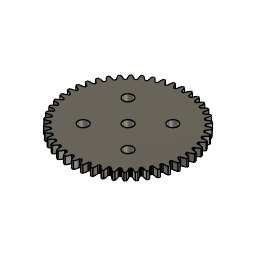
ENGRANAJE_BRAZO (Autodesk Fusion 360 design; units mm, degrees)
description: Spur Gear; Module: 1.0; Num Teeth: 46; Pressure Angle: 20.0; Backlash: 0.00 mm
Autodesk Fusion 360 part; units mm, degrees
sketch "Boceto5" plane through (0, 0, 0) normal (0, 0, 1) x (1, 0, 0)
  line L0 (9, 9) -> (-9, 9) construction
  line L1 (-9, 9) -> (-9, -9) construction
  line L2 (-9, -9) -> (9, -9) construction
  line L3 (9, -9) -> (9, 9) construction
  line L4 (9, 9) -> (-9, -9) construction
  line L5 (-9, 9) -> (9, -9) construction
  circle A0 centre (-9, 9) radius 2
  circle A1 centre (9, 9) radius 2
  circle A2 centre (-9, -9) radius 2
  circle A3 centre (9, -9) radius 2
  dimension "d25" = 4
  dimension "d26" = 4
  dimension "d27" = 4
  dimension "d28" = 4
  constraint horizontal L0
  constraint perpendicular L0 L1
  constraint parallel L0 L2
  constraint parallel L1 L3
  constraint coincident L4 origin
  constraint coincident L5 origin
  constraint coincident L0.end L1.start
  constraint coincident L0.start L3.end
  constraint coincident L1.end L2.start
  constraint coincident L2.end L3.start
  measures "d25" diameter of A0
  measures "d26" diameter of A1
  measures "d27" diameter of A2
  measures "d28" diameter of A3
sketch "Boceto6" plane through (0, 0, 0) normal (0, 0, 1) x (1, 0, 0)
  circle A0 centre (0, 0) radius 21.843
  circle A1 centre (0, 0) radius 2
  dimension "d32" = 4
  measures "d32" diameter of A1
extrude "Extruir4" add sketch "Boceto6" along normal blind 3
sketch "Boceto7" plane through (0, 0, 0) normal (0, 0, 1) x (1, 0, 0)
  spline S0 degree 5 poles (21.5869, -1.0597) (21.5939, -1.0598) (21.6077, -1.0598) (21.6285, -1.0596) (21.6562, -1.0591) (21.6909, -1.0578) (21.7255, -1.0561) (21.7602, -1.0537) (21.7949, -1.0509) (21.8296, -1.0476) (21.8643, -1.0438) (21.899, -1.0397) (21.9337, -1.0353) (21.9684, -1.0305) (22.0031, -1.0255) (22.0378, -1.0202) (22.0725, -1.0147) (22.1071, -1.0088) (22.1418, -1.0027) (22.1765, -0.9963) (22.2112, -0.9897) (22.2458, -0.9828) (22.2805, -0.9757) (22.3151, -0.9684) (22.3498, -0.9608) (22.3844, -0.953) (22.419, -0.945) (22.4536, -0.9368) (22.4882, -0.9284) (22.5228, -0.9198) (22.5574, -0.9109) (22.592, -0.9019) (22.6266, -0.8927) (22.6611, -0.8833) (22.6957, -0.8736) (22.7302, -0.8638) (22.7647, -0.8539) (22.7992, -0.8437) (22.8337, -0.8333) (22.8682, -0.8228) (22.9027, -0.8121) (22.9371, -0.8012) (22.9715, -0.7902) (23.006, -0.7789) (23.0404, -0.7676) (23.0748, -0.756) (23.1092, -0.7443) (23.1435, -0.7324) (23.1779, -0.7203) (23.2122, -0.7081) (23.2465, -0.6957) (23.2808, -0.6832) (23.3151, -0.6705) (23.3494, -0.6576) (23.3836, -0.6446) (23.4179, -0.6315) (23.4521, -0.6181) (23.4863, -0.6047) (23.5204, -0.5911) (23.5546, -0.5773) (23.5888, -0.5634) (23.6229, -0.5493) (23.657, -0.5351) (23.6911, -0.5207) (23.7251, -0.5062) (23.7592, -0.4916) (23.7932, -0.4768) (23.8272, -0.4619) (23.8612, -0.4468) (23.8952, -0.4316) (23.9291, -0.4162) (23.9562, -0.4039) (23.9766, -0.3945) (23.9901, -0.3882) (23.9969, -0.3851) knots 0 0 0 0 0 0 0.01428571 0.02857143 0.04285714 0.05714286 0.07142857 0.08571429 0.1 0.11428571 0.12857143 0.14285714 0.15714286 0.17142857 0.18571429 0.2 0.21428571 0.22857143 0.24285714 0.25714286 0.27142857 0.28571429 0.3 0.31428571 0.32857143 0.34285714 0.35714286 0.37142857 0.38571429 0.4 0.41428571 0.42857143 0.44285714 0.45714286 0.47142857 0.48571429 0.5 0.51428571 0.52857143 0.54285714 0.55714286 0.57142857 0.58571429 0.6 0.61428571 0.62857143 0.64285714 0.65714286 0.67142857 0.68571429 0.7 0.71428571 0.72857143 0.74285714 0.75714286 0.77142857 0.78571429 0.8 0.81428571 0.82857143 0.84285714 0.85714286 0.87142857 0.88571429 0.9 0.91428571 0.92857143 0.94285714 0.95714286 0.97142857 0.98571429 1 1 1 1 1 1
  spline S1 degree 5 poles (21.5869, 1.0597) (21.5939, 1.0598) (21.6077, 1.0598) (21.6285, 1.0596) (21.6562, 1.0591) (21.6909, 1.0578) (21.7255, 1.0561) (21.7602, 1.0537) (21.7949, 1.0509) (21.8296, 1.0476) (21.8643, 1.0438) (21.899, 1.0397) (21.9337, 1.0353) (21.9684, 1.0305) (22.0031, 1.0255) (22.0378, 1.0202) (22.0725, 1.0147) (22.1071, 1.0088) (22.1418, 1.0027) (22.1765, 0.9963) (22.2112, 0.9897) (22.2458, 0.9828) (22.2805, 0.9757) (22.3151, 0.9684) (22.3498, 0.9608) (22.3844, 0.953) (22.419, 0.945) (22.4536, 0.9368) (22.4882, 0.9284) (22.5228, 0.9198) (22.5574, 0.9109) (22.592, 0.9019) (22.6266, 0.8927) (22.6611, 0.8833) (22.6957, 0.8736) (22.7302, 0.8638) (22.7647, 0.8539) (22.7992, 0.8437) (22.8337, 0.8333) (22.8682, 0.8228) (22.9027, 0.8121) (22.9371, 0.8012) (22.9715, 0.7902) (23.006, 0.7789) (23.0404, 0.7676) (23.0748, 0.756) (23.1092, 0.7443) (23.1435, 0.7324) (23.1779, 0.7203) (23.2122, 0.7081) (23.2465, 0.6957) (23.2808, 0.6832) (23.3151, 0.6705) (23.3494, 0.6576) (23.3836, 0.6446) (23.4179, 0.6315) (23.4521, 0.6181) (23.4863, 0.6047) (23.5204, 0.5911) (23.5546, 0.5773) (23.5888, 0.5634) (23.6229, 0.5493) (23.657, 0.5351) (23.6911, 0.5207) (23.7251, 0.5062) (23.7592, 0.4916) (23.7932, 0.4768) (23.8272, 0.4619) (23.8612, 0.4468) (23.8952, 0.4316) (23.9291, 0.4162) (23.9562, 0.4039) (23.9766, 0.3945) (23.9901, 0.3882) (23.9969, 0.3851) knots 0 0 0 0 0 0 0.01428571 0.02857143 0.04285714 0.05714286 0.07142857 0.08571429 0.1 0.11428571 0.12857143 0.14285714 0.15714286 0.17142857 0.18571429 0.2 0.21428571 0.22857143 0.24285714 0.25714286 0.27142857 0.28571429 0.3 0.31428571 0.32857143 0.34285714 0.35714286 0.37142857 0.38571429 0.4 0.41428571 0.42857143 0.44285714 0.45714286 0.47142857 0.48571429 0.5 0.51428571 0.52857143 0.54285714 0.55714286 0.57142857 0.58571429 0.6 0.61428571 0.62857143 0.64285714 0.65714286 0.67142857 0.68571429 0.7 0.71428571 0.72857143 0.74285714 0.75714286 0.77142857 0.78571429 0.8 0.81428571 0.82857143 0.84285714 0.85714286 0.87142857 0.88571429 0.9 0.91428571 0.92857143 0.94285714 0.95714286 0.97142857 0.98571429 1 1 1 1 1 1
  arc A0 (23.9969, -0.3851) -> (23.9969, 0.3851) centre (0, 0) ccw
  line L0 (21.5869, 1.0597) -> (21.5869, -1.0597)
  point P0 (21.7579, -1.0538)
  point P1 (21.9295, -1.0358)
  point P2 (22.1014, -1.0097)
  point P3 (22.2735, -0.9771)
  point P4 (22.4458, -0.9386)
  point P5 (22.6183, -0.8949)
  point P6 (22.7908, -0.8462)
  point P7 (22.9633, -0.7928)
  point P8 (23.1358, -0.735)
  point P9 (23.3083, -0.673)
  point P10 (23.4806, -0.6069)
  point P11 (23.6529, -0.5368)
  point P12 (23.825, -0.4628)
  point P13 (21.7579, 1.0538)
  point P14 (21.9295, 1.0358)
  point P15 (22.1014, 1.0097)
  point P16 (22.2735, 0.9771)
  point P17 (22.4458, 0.9386)
  point P18 (22.6183, 0.8949)
  point P19 (22.7908, 0.8462)
  point P20 (22.9633, 0.7928)
  point P21 (23.1358, 0.735)
  point P22 (23.3083, 0.673)
  point P23 (23.4806, 0.6069)
  point P24 (23.6529, 0.5368)
  point P25 (23.825, 0.4628)
extrude "Extruir5" add sketch "Boceto7" along normal blind 3
fillet "Empalme2" radius 0.4 2 edges at (21.8178, 1.0486, 1.5) (21.8178, -1.0486, 1.5)
pattern_circular "Patrón C2" count 46 over 360 about axis through (0, 0, 0) along (0, 0, 1) of "Extruir5", "Empalme2"
sketch "Boceto8" plane through (0, 0, 0) normal (0, 0, 1) x (1, 0, 0)
  circle A0 centre (0, 0) radius 23 construction
extrude "Extruir6" cut sketch "Boceto5" along normal blind 5
named bodies: "Spur Gear (46 teeth)"
